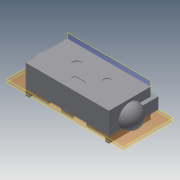
# Autodesk Inventor part: MoistureBeatrobo1
Saved by Autodesk Inventor 2014 (Build 180170000, 170)
## iProperties
Created: 2014-06-14
Part Number: MoistureBeatrobo1
Material: 一般
Document SubType Name: Modeling
Designer: Hideyuki Takei
Density: 1 g/cm^3
Appearance: 既定
Author: Hideyuki Takei
Autodesk Inventor part; units mm, degrees
ref_plane "YZ Plane" through (0, 0, 0) normal (1, 0, 0) x (0, 1, 0)
ref_plane "XZ Plane" through (0, 0, 0) normal (0, 1, 0) x (-1, 0, 0)
sketch "スケッチ1" plane through (0, 0, 0) normal (0, 0, 1) x (1, 0, 0)
  line L0 (0, 20) -> (44, 20)
  line L1 (44, 20) -> (44, -2)
  line L2 (44, -2) -> (0, -2)
  line L3 (0, -2) -> (0, 20)
  point P0 (0, 0)
  dimension "d0" = 44
  dimension "d1" = 22
  dimension "d2" = 20
  dimension "d3" = 0
  constraints: 8 end point, 2 parallel, 1 horizontal, 1 perpendicular
  measures "d0" distance of L0.start L0.end
  measures "d1" distance of L2.end L0.start
  measures "d2" distance from line of point (0, 0) L0
  measures "d3" distance from line of point (0, 0) L3
extrude "押し出し1" add sketch "スケッチ1" along normal blind 15
sketch "スケッチ2" plane through (44, -2, 0) normal (1, 0, 0) x (0, 0, -1)
  line L0 (0, 22) -> (0, 0) projected
  line L1 (0, 0) -> (-15, 0) projected
  circle A0 centre (-7.5, 11) radius 6
  dimension "d6" = 12
  dimension "d7" = 7.5
  dimension "d8" = 11
  constraints: 1 centre point
  measures "d6" diameter of A0
  measures "d7" distance from line of L0 A0.centre
  measures "d8" distance from line of L1 A0.centre
extrude "押し出し2" add sketch "スケッチ2" along normal blind 6
fillet "フィレット1" radius 6 1 edges at (50, 9, 13.5)
sketch "スケッチ3" plane through (0, -2, 0) normal (-1, 0, 0) x (0, 0, 1)
  line L0 (0, 0) -> (0, 22) projected
  line L1 (0, 0) -> (15, 0) projected
  circle A0 centre (7.5, 11) radius 6
  dimension "d12" = 12
  dimension "d13" = 11
  dimension "d14" = 7.5
  constraints: 1 centre point
  measures "d12" diameter of A0
  measures "d13" distance from line of L1 A0.centre
  measures "d14" distance from line of L0 A0.centre
extrude "押し出し3" add sketch "スケッチ3" along normal blind 6
fillet "フィレット2" radius 6 1 edges at (-6, 9, 1.5)
ref_plane "作業平面1" through (0, 22, 0) normal (0, 1, 0) x (1, 0, 0)
sketch "スケッチ5" plane through (0, 22, 0) normal (0, 1, 0) x (1, 0, 0)
  line L0 (0, -4.5) -> (44, -4.5)
  line L1 (44, -4.5) -> (44, -10.5)
  line L2 (44, -10.5) -> (0, -10.5)
  line L3 (0, -10.5) -> (0, -4.5)
  line L4 (0, 0) -> (0, -15) projected
  line L5 (44, -15) -> (0, -15) projected
  dimension "d24" = 44
  dimension "d25" = 6
  dimension "d26" = 0
  dimension "d27" = 4.5
  constraints: 8 end point, 2 parallel, 1 horizontal, 1 perpendicular
  measures "d24" distance of L0.start L0.end
  measures "d25" distance of L2.end L0.start
  measures "d26" distance between parallel lines of L4 L3
  measures "d27" distance between parallel lines of L5 L2
extrude "押し出し5" add sketch "スケッチ5" against normal blind 2
sketch "スケッチ6" plane through (44, -2, 0) normal (1, 0, 0) x (0, 0, -1)
  line L0 (0, 22) -> (0, 0) projected
  line L1 (-10.5, 24) -> (-4.5, 24)
  line L2 (-4.5, 24) -> (-4.5, 12)
  line L3 (-4.5, 12) -> (-10.5, 12)
  line L4 (-10.5, 12) -> (-10.5, 24)
  dimension "d30" = 12
  dimension "d31" = 4.5
  constraints: 8 end point, 2 parallel, 1 horizontal, 1 perpendicular
  measures "d30" distance of L3.end L1.start
  measures "d31" distance between parallel lines of L0 L2
extrude "押し出し6" add sketch "スケッチ6" along normal blind 2
sketch "スケッチ7" plane through (0, -2, 0) normal (-1, 0, 0) x (0, 0, 1)
  line L0 (15, 22) -> (15, 0) projected
  line L1 (4.5, 24) -> (10.5, 24)
  line L2 (10.5, 24) -> (10.5, 12)
  line L3 (10.5, 12) -> (4.5, 12)
  line L4 (4.5, 12) -> (4.5, 24)
  dimension "d34" = 12
  dimension "d35" = 4.5
  constraints: 8 end point, 2 parallel, 1 horizontal, 1 perpendicular
  measures "d34" distance of L3.end L1.start
  measures "d35" distance between parallel lines of L0 L2
extrude "押し出し7" add sketch "スケッチ7" along normal blind 2
sketch "スケッチ8" plane through (0, 0, 0) normal (0, 0, 1) x (1, 0, 0)
  line L0 (42, 18) -> (2, 18)
  line L1 (2, 18) -> (2, 0)
  line L2 (2, 0) -> (42, 0)
  line L3 (42, 0) -> (42, 18)
  line L4 (0, 20) -> (44, 20) projected
  line L5 (44, 20) -> (44, -2) projected
  point P0 (0, 0)
  dimension "d38" = 40
  dimension "d39" = 18
  dimension "d40" = 2
  dimension "d41" = 2
  constraints: 8 end point, 2 parallel, 1 horizontal, 1 perpendicular
  measures "d38" distance of L0.start L0.end
  measures "d39" distance of L2.end L0.start
  measures "d40" distance between parallel lines of L0 L4
  measures "d41" distance between parallel lines of L5 L3
extrude "押し出し8" cut sketch "スケッチ8" along normal blind 13
sketch "スケッチ9" plane through (0, 0, 0) normal (0, 0, 1) x (1, 0, 0)
  line L0 (42, 0) -> (2, 0)
  line L1 (2, 0) -> (2, -2)
  line L2 (2, -2) -> (42, -2)
  line L3 (42, -2) -> (42, 0)
  line L4 (0, 0) -> (0, 20) projected
  line L5 (44, -2) -> (0, -2) projected
  dimension "d44" = 40
  dimension "d45" = 2
  dimension "d46" = 0
  dimension "d47" = 2
  constraints: 8 end point, 2 parallel, 1 horizontal, 1 perpendicular
  measures "d44" distance of L0.start L0.end
  measures "d45" distance between parallel lines of L4 L1
  measures "d46" distance between parallel lines of L5 L2
  measures "d47" distance of L2.end L0.start
extrude "押し出し9" cut sketch "スケッチ9" along normal blind 2
sketch "スケッチ10" plane through (0, 0, 2) normal (0, 0, -1) x (-1, 0, 0)
  line L0 (-42, 0) -> (-2, 0) projected
  line L1 (-42, -2) -> (-42, 0) projected
  line L2 (-2, -2) -> (-42, -2) projected
  line L3 (-18.8, 0) -> (-12, 0)
  line L4 (-12, 0) -> (-12, -2)
  line L5 (-12, -2) -> (-18.8, -2)
  line L6 (-18.8, -2) -> (-18.8, 0)
  line L7 (-2, 18) -> (-2, -2) projected
  line L8 (-25.2, 0) -> (-32, 0)
  line L9 (-32, 0) -> (-32, -2)
  line L10 (-32, -2) -> (-25.2, -2)
  line L11 (-25.2, -2) -> (-25.2, 0)
  point P0 (0, 0)
  dimension "d50" = 6.8
  dimension "d51" = 2
  dimension "d52" = 0
  dimension "d53" = 10
  dimension "d54" = 6.8
  dimension "d55" = 10
  constraints: 16 end point, 4 parallel, 2 horizontal, 2 perpendicular, 2 point on line
  measures "d50" distance of L3.start L3.end
  measures "d51" distance of L5.end L3.start
  measures "d52" distance between parallel lines of L2 L5
  measures "d53" distance between parallel lines of L4 L7
  measures "d54" distance between parallel lines of L11 L9
  measures "d55" distance between parallel lines of L1 L9
extrude "押し出し10" cut sketch "スケッチ10" against normal blind 1.6 contours L0 L11 L2 L9 | L0 L4 L2 L6
fillet "フィレット3" radius 3.3 2 edges at (25.2, 0, 2.8) (18.8, 0, 2.8)
sketch "スケッチ11" plane through (0, 0, 0) normal (0, 0, 1) x (1, 0, 0)
  line L0 (27, 22) -> (17, 22)
  line L1 (17, 22) -> (17, 18)
  line L2 (17, 18) -> (27, 18)
  line L3 (27, 18) -> (27, 22)
  line L4 (44, 20) -> (44, -2) projected
  line L5 (-2, 22) -> (46, 22) projected
  point P0 (0, 0)
  dimension "d59" = 4
  dimension "d60" = 10
  dimension "d61" = 17
  dimension "d62" = 0
  constraints: 8 end point, 2 parallel, 1 horizontal, 1 perpendicular
  measures "d59" distance of L2.end L0.start
  measures "d60" distance of L0.start L0.end
  measures "d61" distance between parallel lines of L3 L4
  measures "d62" distance between parallel lines of L5 L0
extrude "押し出し11" cut sketch "スケッチ11" along normal blind 9.5
ref_plane "作業平面2" through (0, 0, 2) normal (0, 0, 1) x (1, 0, 0)
sketch "スケッチ12" plane through (0, 0, 2) normal (0, 0, 1) x (1, 0, 0)
  line L0 (40, 16) -> (42, 16)
  line L1 (42, 16) -> (42, 18)
  line L2 (42, 18) -> (40, 18)
  line L3 (40, 18) -> (40, 16)
  line L4 (4, 16) -> (2, 16)
  line L5 (2, 16) -> (2, 18)
  line L6 (2, 18) -> (4, 18)
  line L7 (4, 18) -> (4, 16)
  line L8 (42, 18) -> (27, 18) projected
  line L9 (17, 18) -> (2, 18) projected
  line L10 (2, 18) -> (2, -2) projected
  point P0 (0, 0)
  point P1 (42, 0)
  point P2 (41, 18)
  point P3 (3, 18)
  point P4 (2, 17)
  dimension "d66" = 2
  dimension "d67" = 2
  dimension "d68" = 2
  dimension "d69" = 2
  constraints: 16 end point, 4 parallel, 4 point on line, 3 midpoint, 2 horizontal, 2 perpendicular
  measures "d66" distance of L0.start L0.end
  measures "d67" distance of L2.end L0.start
  measures "d68" distance of L6.end L4.start
  measures "d69" distance of L4.start L4.end
extrude "押し出し12" add sketch "スケッチ12" along normal up to next
ref_plane "作業平面3" through (0, 0, 3.6) normal (0, 0, 1) x (1, 0, 0)
sketch "スケッチ13" plane through (0, 0, 3.6) normal (0, 0, 1) x (1, 0, 0)
  line L0 (29, 7) -> (31, 7)
  line L1 (31, 7) -> (31, 10)
  line L2 (31, 10) -> (29, 10)
  line L3 (29, 10) -> (29, 7)
  line L4 (13, 7) -> (15, 7)
  line L5 (15, 7) -> (15, 10)
  line L6 (15, 10) -> (13, 10)
  line L7 (13, 10) -> (13, 7)
  line L8 (42, -2) -> (42, 18) projected
  line L9 (2, 18) -> (2, -2) projected
  line L10 (27, 20) -> (44, 20) projected
  line L11 (0, 20) -> (17, 20) projected
  point P0 (0, 0)
  dimension "d73" = 3
  dimension "d74" = 2
  dimension "d75" = 2
  dimension "d76" = 3
  dimension "d77" = 11
  dimension "d78" = 11
  dimension "d79" = 10
  dimension "d80" = 10
  constraints: 16 end point, 4 parallel, 2 horizontal, 2 perpendicular
  measures "d73" distance of L0.end L1.end
  measures "d74" distance of L0.start L0.end
  measures "d75" distance of L4.start L4.end
  measures "d76" distance of L6.end L4.start
  measures "d77" distance between parallel lines of L8 L1
  measures "d78" distance between parallel lines of L9 L7
  measures "d79" distance between parallel lines of L10 L2
  measures "d80" distance between parallel lines of L6 L11
extrude "押し出し13" add sketch "スケッチ13" along normal up to next
sketch "スケッチ14" plane through (0, 0, 15) normal (0, 0, 1) x (1, 0, 0)
  line L0 (44, 20) -> (0, 20) projected
  line L1 (0, 20) -> (0, -2) projected
  line L2 (44, -2) -> (44, 20) projected
  circle A0 centre (14, 11) radius 2
  circle A1 centre (30, 11) radius 2
  line L3 (19, 5) -> (25, 5)
  line L4 (25, 5) -> (25, 3)
  line L5 (25, 3) -> (19, 3)
  line L6 (19, 3) -> (19, 5)
  line L7 (2, 0) -> (42, 0) projected
  point P0 (0, 0)
  dimension "d83" = 4
  dimension "d84" = 4
  dimension "d85" = 14
  dimension "d86" = 14
  dimension "d87" = 9
  dimension "d88" = 9
  dimension "d91" = 6
  dimension "d92" = 2
  dimension "d93" = 19
  dimension "d94" = 3
  constraints: 8 end point, 2 centre point, 2 parallel, 1 horizontal, 1 perpendicular
  measures "d83" diameter of A0
  measures "d84" diameter of A1
  measures "d85" distance from line of L1 A0.centre
  measures "d86" distance from line of A1.centre L2
  measures "d87" distance from line of L0 A0.centre
  measures "d88" distance from line of L0 A1.centre
  measures "d91" distance of L3.start L3.end
  measures "d92" distance of L5.end L3.start
  measures "d93" distance between parallel lines of L1 L6
  measures "d94" distance between parallel lines of L7 L5
extrude "押し出し14" cut sketch "スケッチ14" against normal blind 0.3
